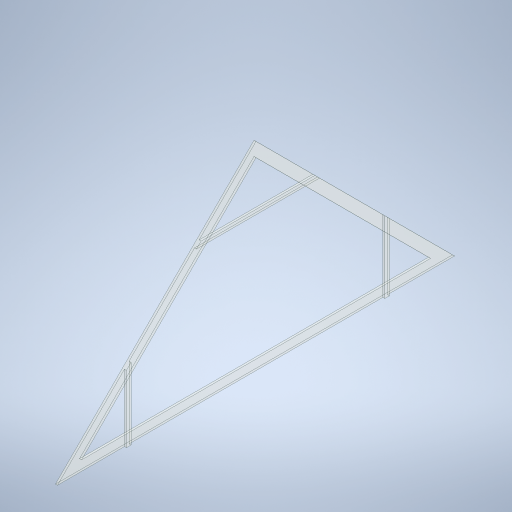
# Autodesk Inventor part: Gable
Saved by Autodesk Inventor 2024 (Build 280153000, 153)
## iProperties
Created: 2023-05-19
Part Number: Gable
Material: Wood (Southern Pine)
Document SubType Name: Modeling
Designer: Tom
Density: 0.420735 g/cm^3
Appearance: Clear
Author: Tom
Autodesk Inventor part; units mm, degrees
ref_plane "YZ Plane" through (0, 0, 0) normal (1, 0, 0) x (0, 1, 0)
ref_plane "XZ Plane" through (0, 0, 0) normal (0, 1, 0) x (-1, 0, 0)
ref_plane "XY Plane" through (0, 0, 0) normal (0, 0, 1) x (1, 0, 0)
sketch "Sketch1" plane through (0, 0, 0) normal (1, 0, 0) x (0, 1, 0)
  line L0 (0, 0) -> (3810, -3810)
  line L1 (3810, -3810) -> (0, -7620)
  line L2 (0, -7620) -> (0, 0)
  line L3 (3540.5923, -3810) -> (190.5, -459.9077)
  line L4 (190.5, -459.9077) -> (190.5, -7160.0923)
  line L5 (190.5, -7160.0923) -> (3540.5923, -3810)
  dimension "d2" = 45
  dimension "d5" = 7620
  dimension "d6" = 190.5
  constraints: 12 end point, 1 perpendicular, 1 vertical, 2 other
  measures "d2" angle of L2 L0
  measures "d5" distance of L1.end L0.start
  measures "d6" distance between parallel lines of L2 L4
extrude "Extrusion1" add sketch "Sketch1" along normal blind 38.1
sketch "Sketch2" plane through (38.1, 0, 0) normal (1, 0, 0) x (0, 0, -1)
  line L0 (3810, 3810) -> (0, 0) projected
  line L1 (2628.9, 2628.9) -> (2717.8, 2717.8)
  line L2 (7620, 0) -> (3810, 3810) projected
  line L3 (4902.2, 2717.8) -> (4991.1, 2628.9)
  line L4 (2628.9, 2628.9) -> (4991.1, 2628.9)
  line L5 (2717.8, 2717.8) -> (4902.2, 2717.8)
  line L6 (459.9077, 190.5) -> (3810, 3540.5923) projected
  line L7 (3810, 3540.5923) -> (7160.0923, 190.5) projected
  line L8 (7160.0923, 190.5) -> (459.9077, 190.5) projected
  line L9 (0, 0) -> (7620, 0) projected
  line L10 (6334.5923, 0) -> (6334.5923, 1285.4077)
  line L11 (6334.5923, 1285.4077) -> (6245.6923, 1374.3077)
  line L12 (6245.6923, 1374.3077) -> (6245.6923, 0)
  line L13 (6245.6923, 0) -> (6334.5923, 0)
  line L14 (1285.4077, 0) -> (1285.4077, 1285.4077)
  line L15 (1285.4077, 1285.4077) -> (1374.3077, 1374.3077)
  line L16 (1374.3077, 1374.3077) -> (1374.3077, 0)
  line L17 (1374.3077, 0) -> (1285.4077, 0)
  point P0 (6245.6923, 1104.9)
  point P1 (6245.6923, 190.5)
  point P2 (1374.3077, 1104.9)
  point P3 (1374.3077, 190.5)
  dimension "d7" = 88.9
  dimension "d9" = 2438.4
  dimension "d10" = 88.9
  dimension "d11" = 914.4
  dimension "d12" = 88.9
  dimension "d14" = 914.4
  constraints: 24 end point, 20 point on line, 3 perpendicular, 2 parallel, 1 collinear, 1 horizontal, 1 vertical
  measures "d7" distance between parallel lines of L4 L5
  measures "d9" distance between parallel lines of L8 L4
  measures "d10" distance between parallel lines of L12 L10
  measures "d11" distance of point (6245.692, 190.5) point (6245.692, 1104.9)
  measures "d12" distance between parallel lines of L16 L14
  measures "d14" distance of point (1374.308, 190.5) point (1374.308, 1104.9)
extrude "Extrusion2" add sketch "Sketch2" along normal blind 38.1 contours L5 L6 L4 L0 | L2 L4 L7 L5 | L5 L7 L4 L6 | L16 L6 L14 L0 | L2 L10 L7 L12 | L16 L8 L14 L6 | L7 L10 L8 L12 | L16 L9 L14 L8 | L8 L10 L9 L12
body "Solid1"
